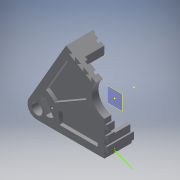
# Autodesk Inventor part: Top_Alpha_V1.1
Saved by Autodesk Inventor 2016 (Build 200138000, 138)
## iProperties
Created: 2015-12-07
Part Number: Top_Alpha_V1.1
Material: Generic
Document SubType Name: Modeling
Designer: Daniel
Density: 1 g/cm^3
Appearance: Default
Mass: 330.234 g
Surface Area: 1237.19 cm^2
Volume: 330.234 cm^3
Author: Daniel
Autodesk Inventor part; units mm, degrees
ref_plane "YZ Plane" through (0, 0, 0) normal (1, 0, 0) x (0, 1, 0)
ref_plane "XZ Plane" through (0, 0, 0) normal (0, 1, 0) x (-1, 0, 0)
ref_plane "XY Plane" through (0, 0, 0) normal (0, 0, 1) x (1, 0, 0)
sketch "Sketch1" plane through (0, 0, 0) normal (0, 1, 0) x (-1, 0, 0)
  circle A0 centre (103.923, -60) radius 8
  circle A1 centre (82.2724, -47.5) radius 2
  line L0 (24.2487, 14) -> (32.909, 19)
  line L1 (36.3731, 21) -> (45.0333, 26)
  line L2 (48.4974, 28) -> (57.1577, 33)
  line L3 (0, -28) -> (0, -38)
  line L4 (0, -42) -> (0, -52)
  line L5 (0, -56) -> (0, -66)
  line L6 (5.1962, -74) -> (103.923, -74)
  arc A2 (103.923, -74) -> (116.0474, -53) centre (103.923, -60) ccw
  line L7 (116.0474, -53) -> (61.4878, 41.5)
  arc A3 (5.1962, -23.4307) -> (17.6935, 16.2154) centre (0, 0) ccw
  line L8 (5.1962, -23.4307) -> (5.1962, -31)
  line L9 (5.1962, -31) -> (0, -28)
  line L10 (0, -28) -> (0, -38)
  line L11 (0, -38) -> (5.1962, -35)
  line L12 (5.1962, -35) -> (5.1962, -45)
  line L13 (5.1962, -45) -> (0, -42)
  line L14 (0, -42) -> (0, -52)
  line L15 (0, -52) -> (5.1962, -49)
  line L16 (5.1962, -49) -> (5.1962, -59)
  line L17 (5.1962, -59) -> (0, -56)
  line L18 (0, -56) -> (0, -66)
  line L19 (0, -66) -> (5.1962, -63)
  line L20 (5.1962, -63) -> (5.1962, -74)
  line L21 (17.6935, 16.2154) -> (24.2487, 20)
  line L22 (24.2487, 20) -> (24.2487, 14)
  line L23 (24.2487, 14) -> (32.909, 19)
  line L24 (32.909, 19) -> (27.7128, 22)
  line L25 (27.7128, 22) -> (36.3731, 27)
  line L26 (36.3731, 27) -> (36.3731, 21)
  line L27 (36.3731, 21) -> (45.0333, 26)
  line L28 (45.0333, 26) -> (39.8372, 29)
  line L29 (39.8372, 29) -> (48.4974, 34)
  line L30 (48.4974, 34) -> (48.4974, 28)
  line L31 (48.4974, 28) -> (57.1577, 33)
  line L32 (57.1577, 33) -> (51.9615, 36)
  line L33 (51.9615, 36) -> (61.4878, 41.5)
  line L34 (91.0088, -29.6319) -> (60.4256, 23.3397)
  line L35 (60.4256, 23.3397) -> (33.1425, 7.5878)
  arc A4 (31.6247, -12.485) -> (33.1425, 7.5878) centre (0, 0) ccw
  line L36 (31.6247, -12.485) -> (78.1742, -39.3604)
  arc A5 (91.0088, -29.6319) -> (78.1742, -39.3604) centre (103.923, -60) ccw
  line L37 (71.1664, -64) -> (15.1962, -64)
  line L38 (15.1962, -64) -> (15.1962, -30.4151)
  arc A6 (15.1962, -30.4151) -> (26.6247, -21.1453) centre (0, 0) ccw
  line L39 (26.6247, -21.1453) -> (73.1742, -48.0206)
  arc A7 (73.1742, -48.0206) -> (71.1664, -64) centre (103.923, -60) ccw
  line L40 (61.4878, 41.5) -> (116.0474, -53)
  line L41 (61.4878, 41.5) -> (51.9615, 36)
  line L42 (57.1577, 33) -> (51.9615, 36)
  line L43 (57.1577, 33) -> (48.4974, 28)
  line L44 (48.4974, 34) -> (48.4974, 28)
  line L45 (48.4974, 34) -> (39.8372, 29)
  line L46 (45.0333, 26) -> (39.8372, 29)
  line L47 (45.0333, 26) -> (36.3731, 21)
  line L48 (36.3731, 21) -> (36.3731, 27)
  line L49 (36.3731, 27) -> (27.7128, 22)
  line L50 (32.909, 19) -> (27.7128, 22)
  line L51 (32.909, 19) -> (24.2487, 14)
  line L52 (24.2487, 14) -> (24.2487, 20)
  line L53 (24.2487, 20) -> (17.6935, 16.2154)
  line L54 (5.1962, -23.4307) -> (5.1962, -31)
  line L55 (0, -28) -> (5.1962, -31)
  line L56 (0, -28) -> (0, -38)
  line L57 (5.1962, -35) -> (0, -38)
  line L58 (5.1962, -35) -> (5.1962, -45)
  line L59 (0, -42) -> (5.1962, -45)
  line L60 (0, -42) -> (0, -52)
  line L61 (0, -52) -> (5.1962, -49)
  line L62 (5.1962, -49) -> (5.1962, -59)
  line L63 (0, -56) -> (5.1962, -59)
  line L64 (0, -56) -> (0, -66)
  line L65 (5.1962, -63) -> (0, -66)
  line L66 (5.1962, -63) -> (5.1962, -74)
  line L67 (5.1962, -74) -> (103.923, -74)
  line L68 (71.1664, -64) -> (15.1962, -64)
  line L69 (15.1962, -64) -> (15.1962, -30.4151)
  line L70 (26.6247, -21.1453) -> (73.1742, -48.0206)
  line L71 (31.6247, -12.485) -> (78.1742, -39.3604)
  line L72 (33.1425, 7.5878) -> (60.4256, 23.3397)
  line L73 (60.4256, 23.3397) -> (91.0088, -29.6319)
  arc A8 (31.6247, -12.485) -> (33.1425, 7.5878) centre (0, 0) ccw
  arc A9 (15.1962, -30.4151) -> (26.6247, -21.1453) centre (0, 0) ccw
  arc A10 (73.1742, -48.0206) -> (71.1664, -64) centre (103.923, -60) ccw
  arc A11 (91.0088, -29.6319) -> (78.1742, -39.3604) centre (103.923, -60) ccw
  arc A12 (5.1962, -23.4307) -> (17.6935, 16.2154) centre (0, 0) ccw
  arc A13 (103.923, -74) -> (116.0474, -53) centre (103.923, -60) ccw
  circle A14 centre (103.923, -60) radius 8
  circle A15 centre (82.2724, -47.5) radius 2
  circle A16 centre (103.923, -60) radius 8
  circle A17 centre (82.2724, -47.5) radius 2
  line L74 (24.2487, 14) -> (32.909, 19)
  line L75 (36.3731, 21) -> (45.0333, 26)
  line L76 (48.4974, 28) -> (57.1577, 33)
  line L77 (0, -28) -> (0, -38)
  line L78 (0, -42) -> (0, -52)
  line L79 (0, -56) -> (0, -66)
  line L80 (5.1962, -74) -> (103.923, -74)
  arc A18 (103.923, -74) -> (116.0474, -53) centre (103.923, -60) ccw
  line L81 (116.0474, -53) -> (61.4878, 41.5)
  arc A19 (5.1962, -23.4307) -> (17.6935, 16.2154) centre (0, 0) ccw
  line L82 (5.1962, -23.4307) -> (5.1962, -31)
  line L83 (5.1962, -31) -> (0, -28)
  line L84 (0, -28) -> (0, -38)
  line L85 (0, -38) -> (5.1962, -35)
  line L86 (5.1962, -35) -> (5.1962, -45)
  line L87 (5.1962, -45) -> (0, -42)
  line L88 (0, -42) -> (0, -52)
  line L89 (0, -52) -> (5.1962, -49)
  line L90 (5.1962, -49) -> (5.1962, -59)
  line L91 (5.1962, -59) -> (0, -56)
  line L92 (0, -56) -> (0, -66)
  line L93 (0, -66) -> (5.1962, -63)
  line L94 (5.1962, -63) -> (5.1962, -74)
  line L95 (17.6935, 16.2154) -> (24.2487, 20)
  line L96 (24.2487, 20) -> (24.2487, 14)
  line L97 (24.2487, 14) -> (32.909, 19)
  line L98 (32.909, 19) -> (27.7128, 22)
  line L99 (27.7128, 22) -> (36.3731, 27)
  line L100 (36.3731, 27) -> (36.3731, 21)
  line L101 (36.3731, 21) -> (45.0333, 26)
  line L102 (45.0333, 26) -> (39.8372, 29)
  line L103 (39.8372, 29) -> (48.4974, 34)
  line L104 (48.4974, 34) -> (48.4974, 28)
  line L105 (48.4974, 28) -> (57.1577, 33)
  line L106 (57.1577, 33) -> (51.9615, 36)
  line L107 (51.9615, 36) -> (61.4878, 41.5)
  line L108 (91.0088, -29.6319) -> (60.4256, 23.3397)
  line L109 (60.4256, 23.3397) -> (33.1425, 7.5878)
  arc A20 (31.6247, -12.485) -> (33.1425, 7.5878) centre (0, 0) ccw
  line L110 (31.6247, -12.485) -> (78.1742, -39.3604)
  arc A21 (91.0088, -29.6319) -> (78.1742, -39.3604) centre (103.923, -60) ccw
  line L111 (71.1664, -64) -> (15.1962, -64)
  line L112 (15.1962, -64) -> (15.1962, -30.4151)
  arc A22 (15.1962, -30.4151) -> (26.6247, -21.1453) centre (0, 0) ccw
  line L113 (26.6247, -21.1453) -> (73.1742, -48.0206)
  arc A23 (73.1742, -48.0206) -> (71.1664, -64) centre (103.923, -60) ccw
  line L114 (61.4878, 41.5) -> (116.0474, -53)
  line L115 (61.4878, 41.5) -> (51.9615, 36)
  line L116 (57.1577, 33) -> (51.9615, 36)
  line L117 (57.1577, 33) -> (48.4974, 28)
  line L118 (48.4974, 34) -> (48.4974, 28)
  line L119 (48.4974, 34) -> (39.8372, 29)
  line L120 (45.0333, 26) -> (39.8372, 29)
  line L121 (45.0333, 26) -> (36.3731, 21)
  line L122 (36.3731, 21) -> (36.3731, 27)
  line L123 (36.3731, 27) -> (27.7128, 22)
  line L124 (32.909, 19) -> (27.7128, 22)
  line L125 (32.909, 19) -> (24.2487, 14)
  line L126 (24.2487, 14) -> (24.2487, 20)
  line L127 (24.2487, 20) -> (17.6935, 16.2154)
  line L128 (5.1962, -23.4307) -> (5.1962, -31)
  line L129 (0, -28) -> (5.1962, -31)
  line L130 (0, -28) -> (0, -38)
  line L131 (5.1962, -35) -> (0, -38)
  line L132 (5.1962, -35) -> (5.1962, -45)
  line L133 (0, -42) -> (5.1962, -45)
  line L134 (0, -42) -> (0, -52)
  line L135 (0, -52) -> (5.1962, -49)
  line L136 (5.1962, -49) -> (5.1962, -59)
  line L137 (0, -56) -> (5.1962, -59)
  line L138 (0, -56) -> (0, -66)
  line L139 (5.1962, -63) -> (0, -66)
  line L140 (5.1962, -63) -> (5.1962, -74)
  line L141 (5.1962, -74) -> (103.923, -74)
  line L142 (71.1664, -64) -> (15.1962, -64)
  line L143 (15.1962, -64) -> (15.1962, -30.4151)
  line L144 (26.6247, -21.1453) -> (73.1742, -48.0206)
  line L145 (31.6247, -12.485) -> (78.1742, -39.3604)
  line L146 (33.1425, 7.5878) -> (60.4256, 23.3397)
  line L147 (60.4256, 23.3397) -> (91.0088, -29.6319)
  arc A24 (31.6247, -12.485) -> (33.1425, 7.5878) centre (0, 0) ccw
  arc A25 (15.1962, -30.4151) -> (26.6247, -21.1453) centre (0, 0) ccw
  arc A26 (73.1742, -48.0206) -> (71.1664, -64) centre (103.923, -60) ccw
  arc A27 (91.0088, -29.6319) -> (78.1742, -39.3604) centre (103.923, -60) ccw
  arc A28 (5.1962, -23.4307) -> (17.6935, 16.2154) centre (0, 0) ccw
  arc A29 (103.923, -74) -> (116.0474, -53) centre (103.923, -60) ccw
  circle A30 centre (103.923, -60) radius 8
  circle A31 centre (82.2724, -47.5) radius 2
  point P0 (0, 0)
  point P1 (0, 0)
  constraints: 296 end point, 48 point on circle, 44 collinear, 32 centre point, 18 parallel, 12 point on line, 10 concentric, 4 coincident, 4 perpendicular, 4 tangent
ref_plane "Plano de trabajo2" through (0, 10, 0) normal (0, 1, 0) x (1, 0, 0)
sketch "Boceto8" plane through (0, 10, 0) normal (0, 1, 0) x (1, 0, 0)
  line L0 (-116.0474, 53) -> (-61.4878, -41.5) projected
  arc A0 (-103.923, 74) -> (-116.0474, 53) centre (-103.923, 60) ccw projected
  line L1 (-5.1962, 74) -> (-103.923, 74) projected
  line L2 (-5.1962, 63) -> (-5.1962, 74) projected
  line L3 (0, 66) -> (-5.1962, 63) projected
  line L4 (0, 56) -> (0, 66) projected
  line L5 (-5.1962, 59) -> (0, 56) projected
  line L6 (-61.4878, -41.5) -> (-51.9615, -36) projected
  line L7 (-51.9615, -36) -> (-57.1577, -33) projected
  line L8 (-57.1577, -33) -> (-48.4974, -28) projected
  line L9 (-5.1962, 49) -> (-5.1962, 59) projected
  line L10 (-48.4974, -28) -> (-48.4974, -34) projected
  arc A1 (-103.923, 71) -> (-113.4493, 54.5) centre (-103.923, 60) ccw
  line L11 (-113.4493, 54.5) -> (-63.9878, -31.1699)
  line L12 (-63.9878, -31.1699) -> (-43.4974, -19.3397)
  line L13 (-10.1962, 71) -> (-103.923, 71)
  line L14 (-43.4974, -19.3397) -> (-43.4974, -31.1132)
  line L15 (-5.1962, 49) -> (-10.1962, 49)
  line L16 (-10.1962, 49) -> (-10.1962, 71)
  line L17 (-48.4974, -34) -> (-43.4974, -31.1132)
  point P0 (0, 0)
  dimension "d41" = 3
  dimension "d44" = 5
  dimension "d45" = 5
  dimension "d49" = 5
  constraints: 14 end point, 4 parallel, 2 point on circle, 2 tangent, 1 centre point, 1 coincident, 1 collinear, 1 horizontal, 1 perpendicular
  measures "d41" radial gap between concentric circles of A0 A1
  measures "d44" distance between parallel lines of L12 L8
  measures "d45" distance between parallel lines of L10 L14
  measures "d49" distance between parallel lines of L9 L16
extrude "Extrusión13" add sketch "Sketch1" along normal blind 5
sketch "Boceto11" plane through (0, 5, 0) normal (0, 1, 0) x (1, 0, 0)
  line L0 (-60.4256, -23.3397) -> (-91.0088, 29.6319) projected
  arc A0 (-91.0088, 29.6319) -> (-78.1742, 39.3604) centre (-103.923, 60) ccw projected
  line L1 (-78.1742, 39.3604) -> (-31.6247, 12.485) projected
  arc A1 (-31.6247, 12.485) -> (-33.1425, -7.5878) centre (0, 0) ccw projected
  line L2 (-33.1425, -7.5878) -> (-60.4256, -23.3397) projected
  line L3 (-15.1962, 64) -> (-15.1962, 30.4151) projected
  arc A2 (-15.1962, 30.4151) -> (-26.6247, 21.1453) centre (0, 0) ccw projected
  line L4 (-26.6247, 21.1453) -> (-73.1742, 48.0206) projected
  arc A3 (-73.1742, 48.0206) -> (-71.1664, 64) centre (-103.923, 60) ccw projected
  line L5 (-71.1664, 64) -> (-15.1962, 64) projected
  circle A4 centre (-103.923, 60) radius 8 projected
  circle A5 centre (-82.2724, 47.5) radius 2 projected
  arc A6 (-103.923, 74) -> (-116.0474, 53) centre (-103.923, 60) ccw projected
  line L6 (-116.0474, 53) -> (-61.4878, -41.5) projected
  line L7 (-61.4878, -41.5) -> (-51.9615, -36) projected
  line L8 (-51.9615, -36) -> (-57.1577, -33) projected
  line L9 (-57.1577, -33) -> (-48.4974, -28) projected
  line L10 (-48.4974, -28) -> (-48.4974, -34) projected
  line L11 (-48.4974, -34) -> (-39.8372, -29) projected
  line L12 (-39.8372, -29) -> (-45.0333, -26) projected
  line L13 (-45.0333, -26) -> (-36.3731, -21) projected
  line L14 (-36.3731, -21) -> (-36.3731, -27) projected
  line L15 (-36.3731, -27) -> (-27.7128, -22) projected
  line L16 (-27.7128, -22) -> (-32.909, -19) projected
  line L17 (-32.909, -19) -> (-24.2487, -14) projected
  line L18 (-24.2487, -14) -> (-24.2487, -20) projected
  line L19 (-24.2487, -20) -> (-17.6935, -16.2154) projected
  arc A7 (-5.1962, 23.4307) -> (-17.6935, -16.2154) centre (0, 0) ccw projected
  line L20 (-5.1962, 23.4307) -> (-5.1962, 31) projected
  line L21 (-5.1962, 31) -> (0, 28) projected
  line L22 (0, 28) -> (0, 38) projected
  line L23 (0, 38) -> (-5.1962, 35) projected
  line L24 (-5.1962, 35) -> (-5.1962, 45) projected
  line L25 (-5.1962, 45) -> (0, 42) projected
  line L26 (0, 42) -> (0, 52) projected
  line L27 (0, 52) -> (-5.1962, 49) projected
  line L28 (-5.1962, 49) -> (-5.1962, 59) projected
  line L29 (-5.1962, 59) -> (0, 56) projected
  line L30 (0, 56) -> (0, 66) projected
  line L31 (0, 66) -> (-5.1962, 63) projected
  line L32 (-5.1962, 63) -> (-5.1962, 74) projected
  line L33 (-5.1962, 74) -> (-103.923, 74) projected
  point P0 (0, 0)
extrude "Extrusión14" add sketch "Boceto11" along normal blind 5 contours L0 A0 L1 A1 L2 | L3 A2 L4 A3 L5 | L33 L32 L31 L30 L29 L28 L27 L26 L25 L24 L23 L22 L21 L20 A7 L19 L18 L17 L16 L15 L14 L13 L12 L11 L10 L9 L8 L7 L6 A6
extrude "Extrusión15" add sketch "Boceto8" along normal blind 30
sketch "Boceto22" plane through (0, 10, 0) normal (0, 1, 0) x (1, 0, 0)
  circle A0 centre (-103.923, 60) radius 8 projected
  arc A1 (-103.923, 74) -> (-116.0474, 53) centre (-103.923, 60) ccw
  arc A2 (-103.923, 71) -> (-113.4493, 54.5) centre (-103.923, 60) ccw projected
  line L0 (-10.1962, 71) -> (-103.923, 71) projected
  arc A3 (-98.0749, 27.8707) -> (-73.1742, 71) centre (-103.923, 60) ccw
  line L1 (-113.4493, 54.5) -> (-63.9878, -31.1699) projected
  line L2 (-113.4493, 54.5) -> (-98.0749, 27.8707)
  line L3 (-116.0474, 53) -> (-61.4878, -41.5) projected
  line L4 (-103.923, 71) -> (-73.1742, 71)
  line L5 (-5.1962, 74) -> (-103.923, 74) projected
  line L6 (-98.0749, 27.8707) -> (-73.1742, 71)
  line L7 (-99.8069, 30.8707) -> (-76.6383, 71)
  line L8 (-99.8069, 30.8707) -> (-98.0749, 27.8707)
  line L9 (-76.6383, 71) -> (-73.1742, 71)
  point P0 (0, 0)
  dimension "d76" = 3
  constraints: 12 end point, 4 point on circle, 3 parallel, 3 point on line, 2 centre point, 1 coincident, 1 collinear
  measures "d76" distance between parallel lines of L6 L7
extrude "Extrusión21" add sketch "Boceto22" along normal blind 2.5 contours L0 L6 L1 L7 | A3 L6
sketch "Boceto23" plane through (0, 12.5, 0) normal (0, 1, 0) x (1, 0, 0)
  line L0 (-76.6383, 71) -> (-73.1742, 71) projected
  line L1 (-76.6383, 71) -> (-99.8069, 30.8707) projected
  line L2 (-98.0749, 27.8707) -> (-99.8069, 30.8707) projected
  line L3 (-73.1742, 71) -> (-98.0749, 27.8707)
  point P0 (0, 0)
  constraints: 2 end point
extrude "Extrusión22" add sketch "Boceto23" along normal blind 25.5
sketch "Boceto25" plane through (0, 10, 0) normal (0, 1, 0) x (1, 0, 0)
  circle A0 centre (-103.923, 60) radius 8 projected
  circle A1 centre (-103.923, 60) radius 8 projected
  line L0 (-99.8069, 30.8707) -> (-76.6383, 71) projected
  arc A2 (-103.923, 71) -> (-113.4493, 54.5) centre (-103.923, 60) ccw
  line L1 (-113.4493, 54.5) -> (-104.5004, 39)
  line L2 (-113.4493, 54.5) -> (-99.8069, 30.8707) projected
  line L3 (-103.923, 71) -> (-86.0252, 71)
  line L4 (-76.6383, 71) -> (-103.923, 71) projected
  line L5 (-104.5004, 39) -> (-86.0252, 71)
  point P0 (0, 0)
  dimension "d110" = 10
  constraints: 6 end point, 2 point on circle, 2 point on line, 1 centre point, 1 coincident, 1 parallel
  measures "d110" distance from line of A0.centre L5
extrude "Extrusión23" add sketch "Boceto25" along normal blind 20 contours L1 A2 L3 L5
sketch "Boceto26" plane through (0, 30, 0) normal (0, 1, 0) x (1, 0, 0)
  arc A0 (-103.923, 71) -> (-113.4493, 54.5) centre (-103.923, 60) ccw projected
  line L0 (-104.5004, 39) -> (-113.4493, 54.5) projected
  line L1 (-104.5004, 39) -> (-86.0252, 71) projected
  circle A1 centre (-103.923, 60) radius 8 projected
  line L2 (-103.923, 71) -> (-86.0252, 71) projected
  point P0 (0, 0)
extrude "Extrusión24" add sketch "Boceto26" along normal blind 8 contours L2 L1 L0 A0 | A1
sketch "Boceto29" plane through (0, 40, 0) normal (0, 1, 0) x (1, 0, 0)
  line L0 (-10.1962, 71) -> (-10.1962, 49) projected
  line L1 (-10.1962, 49) -> (-5.1962, 49) projected
  line L2 (-5.1962, 49) -> (-5.1962, 59) projected
  line L3 (-5.1962, 59) -> (0, 56) projected
  line L4 (0, 56) -> (0, 66) projected
  line L5 (0, 66) -> (-5.1962, 63) projected
  line L6 (-5.1962, 63) -> (-5.1962, 74) projected
  line L7 (-5.1962, 74) -> (-103.923, 74) projected
  line L8 (-103.923, 71) -> (-10.1962, 71) projected
  line L9 (-10.1962, 71) -> (-5.1962, 71)
  line L10 (-43.4974, -31.1132) -> (-43.4974, -19.3397) projected
  line L11 (-48.4974, -34) -> (-43.4974, -31.1132) projected
  line L12 (-48.4974, -28) -> (-48.4974, -34) projected
  line L13 (-57.1577, -33) -> (-48.4974, -28) projected
  line L14 (-51.9615, -36) -> (-57.1577, -33) projected
  line L15 (-61.4878, -41.5) -> (-51.9615, -36) projected
  line L16 (-43.4974, -19.3397) -> (-63.9878, -31.1699) projected
  line L17 (-63.9878, -31.1699) -> (-58.8897, -40)
  point P0 (0, 0)
  constraints: 4 end point, 2 perpendicular, 2 point on line
extrude "Extrusión25" cut sketch "Boceto29" against normal blind 2
sketch "Boceto30" plane through (-73.1742, 12.5, -71) normal (0.8660254, 0, 0.5) x (0.5, 0, -0.8660254)
  circle A0 centre (-9.4007, 13) radius 1.7068
  circle A1 centre (-40.4007, 13) radius 1.9288
  line L0 (-9.4007, 13) -> (-40.4007, 13) construction
  line L1 (0, 0) -> (-49.8015, 0) projected
  line L2 (-9.4007, 13) -> (0, 13) construction
  line L3 (0, 25.5) -> (0, 0) projected
  line L4 (-40.4007, 13) -> (-49.8015, 13) construction
  line L5 (-49.8015, 0) -> (-49.8015, 25.5) projected
  line L6 (-49.8015, 25.5) -> (0, 25.5) projected
  arc A2 (-36.4007, 13) -> (-39.0998, 16.7825) centre (-40.4007, 13) ccw
  arc A3 (-10.7017, 16.7825) -> (-13.4007, 13) centre (-9.4007, 13) ccw
  arc A4 (-49.8015, 25.5) -> (-39.0998, 16.7825) centre (-32.5951, 35.6952) ccw
  line L7 (-36.4007, 13) -> (-36.4007, 0)
  arc A5 (-10.7017, 16.7825) -> (0, 25.5) centre (-17.2063, 35.6952) ccw
  line L8 (-13.4007, 13) -> (-13.4007, 0)
  point P0 (-24.9007, -12.5)
  dimension "d94" = 31
  dimension "d99" = 4
  dimension "d100" = 4
  dimension "d101" = 20
  dimension "d102" = 20
  dimension "d105" = 13
  constraints: 10 end point, 8 point on circle, 6 centre point, 6 point on line, 2 coincident, 2 horizontal, 2 perpendicular, 2 tangent, 1 collinear, 1 parallel
  measures "d94" distance of L0.start L0.end
  measures "d99" radius of A2
  measures "d100" radius of A3
  measures "d101" radius of A4
  measures "d102" radius of A5
  measures "d105" distance from line of L1 L0.end
extrude "Extrusión26" cut sketch "Boceto30" against normal up to surface (3 mm away) contours A0 | A1 | L1 L7 A2 A4 L6 A5 A3 L8
sketch "Boceto32" plane through (0, 10, 0) normal (0, 1, 0) x (1, 0, 0)
  line L0 (-86.0252, 71) -> (-104.5004, 39) projected
  line L1 (-104.5004, 39) -> (-99.8069, 30.8707) projected
  line L2 (-99.8069, 30.8707) -> (-76.6383, 71) projected
  line L3 (-76.6383, 71) -> (-86.0252, 71) projected
  point P0 (0, 0)
extrude "Extrusión27" add sketch "Boceto32" along normal blind 2.5
sketch "Boceto33" plane through (0, 12.5, 0) normal (0, 1, 0) x (1, 0, 0)
  line L0 (-73.1742, 71) -> (-79.8745, 59.3946) projected
  line L1 (-79.8745, 59.3946) -> (-82.4726, 60.8946) projected
  line L2 (-76.6383, 71) -> (-82.4726, 60.8946) projected
  line L3 (-86.0252, 71) -> (-76.6383, 71) projected
  line L4 (-104.5004, 39) -> (-86.0252, 71) projected
  line L5 (-99.8069, 30.8707) -> (-104.5004, 39) projected
  line L6 (-93.9726, 40.976) -> (-99.8069, 30.8707) projected
  line L7 (-91.3745, 39.476) -> (-93.9726, 40.976) projected
  line L8 (-91.3745, 39.476) -> (-98.0749, 27.8707) projected
  arc A0 (-98.0749, 27.8707) -> (-73.1742, 71) centre (-103.923, 60) ccw projected
  line L9 (-91.3745, 39.476) -> (-79.8745, 59.3946)
  line L10 (-91.3745, 39.476) -> (-93.9726, 40.976) projected
  line L11 (-93.9726, 40.976) -> (-82.4726, 60.8946) construction
  arc A1 (-82.4726, 60.8946) -> (-91.1957, 62.0444) centre (-88.2226, 50.9353) ccw
  arc A2 (-99.3299, 47.9556) -> (-93.9726, 40.976) centre (-88.2226, 50.9353) ccw
  line L12 (-99.3299, 47.9556) -> (-91.1957, 62.0444)
  point P0 (0, 0)
  constraints: 6 end point, 4 point on circle, 2 centre point, 2 collinear, 1 coincident, 1 midpoint, 1 perpendicular, 1 point on line
extrude "Extrusión29" cut sketch "Boceto33" against normal up to next contours L9 L7 A2 L4 A1 L1
sketch "Boceto41" plane through (0, 38, 0) normal (0, 1, 0) x (1, 0, 0)
  arc A0 (-103.923, 71) -> (-113.4493, 54.5) centre (-103.923, 60) ccw projected
  line L0 (-103.923, 60) -> (-113.4493, 65.5) construction
  circle A1 centre (-103.923, 60) radius 8 projected
  line L1 (-116.0474, 53) -> (-61.4878, -41.5) projected
  circle A2 centre (-103.923, 60) radius 1.5
  point P0 (0, 0)
  dimension "d121" = 3
  constraints: 2 end point, 1 centre point, 1 coincident, 1 point on circle
  measures "d121" diameter of A2
extrude "Extrusión30" cut sketch "Boceto41" against normal up to next contours A2
sketch "Boceto44" plane through (-86.0252, 12.5, -71) normal (0.8660254, 0, 0.5) x (0.5, 0, -0.8660254)
  line L0 (-36.9504, 25.5) -> (0, 25.5) projected
  line L1 (-18.4752, 25.5) -> (-18.4752, 17.5) construction
  line L2 (-26.4752, 17.5) -> (-10.4752, 17.5) projected
  line L3 (-21.2252, 23) -> (-15.7252, 23)
  line L4 (-15.7252, 23) -> (-15.7252, 20.6)
  line L5 (-15.7252, 20.6) -> (-21.2252, 20.6)
  line L6 (-21.2252, 20.6) -> (-21.2252, 23)
  point P0 (-18.4752, -12.5)
  dimension "d124" = 5.5
  dimension "d125" = 2.4
  dimension "d126" = 2.5
  constraints: 10 end point, 2 midpoint, 2 parallel, 1 horizontal, 1 perpendicular, 1 symmetric about line, 1 vertical
  measures "d124" distance of L4.end L5.end
  measures "d125" distance of L5.end L3.start
  measures "d126" distance between parallel lines of L0 L3
extrude "Extrusión31" cut sketch "Boceto44" against normal blind 13.175
sketch "Boceto46" plane through (0, 10, 0) normal (0, 1, 0) x (1, 0, 0)
  line L0 (-10.1962, 61.7629) -> (25.1866, 76.3843)
  point P0 (0, 0)
  point P1 (0, 66)
  constraints: 2 end point
sketch "Boceto47" plane through (-10.1962, 10, -71) normal (-1, 0, 0) x (0, 0, 1)
  line L0 (22, 0) -> (0, 0) projected
  line L1 (8, -10) -> (8, 28) projected
  line L2 (8, 28) -> (8, 0)
  line L3 (0, 0) -> (0, 28) projected
  line L4 (8, 28) -> (0, 28)
  line L5 (0, 28) -> (0, 0)
  line L6 (0, 0) -> (8, 0)
  point P0 (71, -10)
  constraints: 8 end point, 2 point on line, 1 collinear, 1 horizontal, 1 perpendicular
extrude "Extrusión32" add sketch "Boceto47" along normal blind 5
sketch "Boceto51" plane through (0, 38, 0) normal (0, 1, 0) x (1, 0, 0)
  circle A0 centre (-10.1962, 67) radius 1.5
  line L0 (-15.1962, 63) -> (-15.1962, 71) projected
  line L1 (-15.1962, 67) -> (-10.1962, 67) construction
  line L2 (-10.1962, 63) -> (-10.1962, 67) construction
  point P0 (0, 0)
  dimension "d136" = 3
  constraints: 4 end point, 1 centre point, 1 coincident, 1 midpoint, 1 perpendicular, 1 vertical
  measures "d136" diameter of A0
extrude "Extrusión33" cut sketch "Boceto51" against normal blind 25
sketch "Boceto52" plane through (-15.1962, 10, -71) normal (-1, 0, 0) x (0, 0, 1)
  line L0 (0.825, 26) -> (7.175, 26)
  line L1 (7.175, 26) -> (7.175, 23.5)
  line L2 (7.175, 23.5) -> (0.825, 23.5)
  line L3 (0.825, 23.5) -> (0.825, 26)
  line L4 (8, 28) -> (0, 28) projected
  line L5 (4, 28) -> (4, 16.5464) construction
  point P0 (71, -10)
  dimension "d139" = 6.35
  dimension "d140" = 2.5
  dimension "d141" = 2
  constraints: 10 end point, 2 parallel, 1 horizontal, 1 midpoint, 1 perpendicular, 1 symmetric about line, 1 vertical
  measures "d139" distance of L1.end L2.end
  measures "d140" distance of L0.end L1.end
  measures "d141" distance between parallel lines of L0 L4
extrude "Extrusión34" cut sketch "Boceto52" against normal blind 8.2
sketch "Boceto53" plane through (-43.4974, 10, 19.3397) normal (-0.5, 0, -0.8660254) x (-0.8660254, 0, 0.5)
  line L0 (23.6603, 28) -> (0, 28) projected
  line L1 (23.6603, 28) -> (15.6603, 28)
  line L2 (15.6603, 28) -> (15.6603, 0)
  line L3 (15.6603, 0) -> (23.6603, 0)
  line L4 (23.6603, 0) -> (23.6603, 28) projected
  line L5 (23.6603, 0) -> (23.6603, 28)
  point P0 (-47.3397, -10)
  dimension "d144" = 8
  constraints: 8 end point, 3 perpendicular, 1 point on line
  measures "d144" distance of L0.start L1.end
extrude "Extrusión35" add sketch "Boceto53" along normal blind 5
sketch "Boceto54" plane through (0, 38, 0) normal (0, 1, 0) x (1, 0, 0)
  line L0 (-57.0596, -27.1699) -> (-43.4974, -19.3397) projected
  line L1 (-57.0596, -27.1699) -> (-60.097, -28.9235)
  line L2 (-116.0474, 53) -> (-61.4878, -41.5) projected
  point P0 (0, 0)
  constraints: 2 end point, 1 perpendicular
